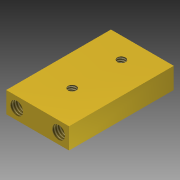
# Autodesk Inventor part: 13_0204_066
Saved by Autodesk Inventor 2012 SP1 (Build 160190100, 190)
## iProperties
Created: 2013-04-30
Part Number: 13_0204_066
Material: Default
Document SubType Name: Modeling
Designer: vogel
Density: 1 g/cm^3
Author: vogel
Autodesk Inventor part; units mm, degrees
ref_plane "YZ Plane" through (0, 0, 0) normal (1, 0, 0) x (0, 1, 0)
ref_plane "XZ Plane" through (0, 0, 0) normal (0, 1, 0) x (-1, 0, 0)
ref_plane "XY Plane" through (0, 0, 0) normal (0, 0, 1) x (1, 0, 0)
sketch "Skizze1" plane through (0, 0, 0) normal (0, 0, 1) x (1, 0, 0)
  line L0 (0, 0) -> (12, 0)
  line L1 (12, 0) -> (12, 20)
  line L2 (12, 20) -> (0, 20)
  line L3 (0, 20) -> (0, 0)
  dimension "d0" = 20
  dimension "d1" = 12
  constraints: 8 end point, 2 parallel, 1 horizontal, 1 perpendicular
  measures "d0" distance of L2.end L0.start
  measures "d1" distance of L0.start L0.end
extrude "Extrusion1" add sketch "Skizze1" along normal blind 4
sketch "Skizze2" plane through (0, 0, 0) normal (0, -1, 0) x (1, 0, 0)
  line L0 (12, 4) -> (0, 4) projected
  line L1 (0, 0) -> (0, 4) projected
  line L2 (0, 0) -> (12, 0) projected
  line L3 (12, 0) -> (12, 4) projected
  line L4 (0, 2) -> (12, 2)
  line L5 (6, 4) -> (6, 0)
  point P0 (2, 2)
  point P1 (10, 2)
  dimension "d4" = 8
  constraints: 4 end point, 4 midpoint, 2 point on line, 1 symmetric about line
  measures "d4" distance of point (10, 2) point (2, 2)
hole "Bohrung1" at (2, 0, 2) at (10, 0, 2) direction (0, 1, 0) diameter 2.459 depth 10 tip angle 118 thread size "M3x0.5" class "6H" standard "ISO Metric profile"
sketch "Skizze3" plane through (0, 0, 4) normal (0, 0, 1) x (1, 0, 0)
  line L0 (12, 0) -> (0, 0) projected
  line L1 (0, 20) -> (12, 20) projected
  line L2 (6, 0) -> (6, 20)
  point P0 (6, 16)
  point P1 (6, 6.6)
  dimension "d13" = 9.4
  dimension "d14" = 4
  constraints: 2 end point, 2 midpoint, 2 point on line
  measures "d13" distance of point (6, 6.6) point (6, 16)
  measures "d14" distance from line of L1 point (6, 16)
hole "Bohrung2" at (6, 16, 4) at (6, 6.6, 4) direction (0, 0, -1) diameter 1.567 depth 10 tip angle 118 thread size "M2x0.4" class "6H" standard "ISO Metric profile"
